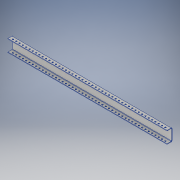
# Autodesk Inventor part: Intake front inner
Saved by Autodesk Inventor 2019 (Build 230136000, 136)
## iProperties
Created: 2018-11-07
Part Number: Intake front inner
Material: Aluminum 6061
Document SubType Name: Sheet Metal
Designer: woodk
Density: 2.7 g/cm^3
Sheet Metal Rule: Haakon
Appearance: Aluminum - Flat
Mass: 253.541 g
Surface Area: 982.103 cm^2
Volume: 93.904 cm^3
Author: woodk
Autodesk Inventor part; units mm, degrees
ref_plane "YZ Plane" through (0, 0, 0) normal (1, 0, 0) x (0, 1, 0)
ref_plane "XZ Plane" through (0, 0, 0) normal (0, 1, 0) x (-1, 0, 0)
ref_plane "XY Plane" through (0, 0, 0) normal (0, 0, 1) x (1, 0, 0)
sketch "Sketch1" plane through (0, 0, 0) normal (0, 0, 1) x (1, 0, 0)
  line L0 (0, 0) -> (609.6, 0)
  line L1 (609.6, 0) -> (609.6, 46.736)
  line L2 (609.6, 46.736) -> (0, 46.736)
  line L3 (0, 46.736) -> (0, 0)
  dimension "d0" = 46.736
  dimension "d1" = 609.6
  measures "d0" distance of L2.end L0.start
  measures "d1" distance of L0.start L0.end
extrude "Plate1" add sketch "Sketch1" along normal blind 2.032
sketch "Sketch2" plane through (0, 44.704, 0) normal (0, 1, 0) x (-1, 0, 0)
  line L0 (-609.6, 0) -> (0, 0)
  line L1 (0, 0) -> (0, 19.05)
  line L2 (0, 19.05) -> (-609.6, 19.05)
  line L3 (-609.6, 19.05) -> (-609.6, 0)
  constraints: 6 end point, 1 horizontal, 1 perpendicular, 1 vertical
edge flange "Flange1" height 19.05 angle 90 thickness 2.032 bend radius 1.27 thickness toward (0, 1, 0) relief tear relief width 2.032 relief depth 1.016 edges at (304.8, 46.736, 2.032) wall of the first edge with corners at (609.6, 44.704, 0) (0, 44.704, 0) (0, 44.704, 19.05) (609.6, 44.704, 19.05)
bend "Bend1"
corner "Corner1"
sketch "Sketch3" plane through (609.6, 2.032, 0) normal (0, -1, 0) x (1, 0, 0)
  line L0 (-609.6, 0) -> (0, 0)
  line L1 (0, 0) -> (0, 19.05)
  line L2 (0, 19.05) -> (-609.6, 19.05)
  line L3 (-609.6, 19.05) -> (-609.6, 0)
  constraints: 6 end point, 1 horizontal, 1 perpendicular, 1 vertical
edge flange "Flange2" height 19.05 angle 90 thickness 2.032 bend radius 1.27 thickness toward (0, -1, 0) relief tear relief width 2.032 relief depth 1.016 edges at (304.8, 0, 2.032) wall of the first edge with corners at (0, 2.032, 0) (609.6, 2.032, 0) (609.6, 2.032, 19.05) (0, 2.032, 19.05)
bend "Bend2"
corner "Corner2"
sketch "Sketch4" plane through (0, 46.736, 19.05) normal (0, 1, 0) x (1, 0, 0)
  line L0 (0, 0) -> (0, 15.748) projected
  line L1 (0, 19.05) -> (609.6, 19.05) projected
  point P0 (12.7, 6.35)
  dimension "d23" = 12.7
  dimension "d24" = 12.7
  measures "d23" distance from line of L0 point (12.7, 6.35)
  measures "d24" distance from line of L1 point (12.7, 6.35)
hole "Hole1" at (12.7, 46.736, 12.7) direction (0, -1, 0) diameter 4.9784 end through all
pattern_linear "Rectangular Pattern1" count 47 spacing 12.7 along (1, 0, 0) of "Hole1"
equation "\"d30\" = Thickness"
equation "\"d2\" = Thickness"
equation "\"d3\" = BendReliefWidth"
equation "\"d4\" = BendReliefDepth"
equation "\"d5\" = MinimumRemnant"
equation "\"d6\" = TransitionRadius"
equation "\"d9\" = BendRadius"
equation "\"d10\" = CornerReliefSize"
equation "\"d11\" = GapSize"
equation "\"d12\" = JacobiRadiusSize"
equation "\"d13\" = BendReliefWidth"
equation "\"d14\" = BendReliefDepth"
equation "\"d15\" = MinimumRemnant"
equation "\"d16\" = TransitionRadius"
equation "\"d19\" = BendRadius"
equation "\"d20\" = CornerReliefSize"
equation "\"d21\" = GapSize"
equation "\"d22\" = JacobiRadiusSize"
equation "\"BendReliefWidth\" = Thickness"
equation "\"BendReliefDepth\" = 0.5 * Thickness"
equation "\"CornerReliefSize\" = 4 * Thickness"
equation "\"MinimumRemnant\" = 2 * Thickness"
equation "\"TransitionRadius\" = BendRadius"
equation "\"JacobiRadiusSize\" = BendRadius"
equation "\"GapSize\" = Thickness"
equation "\"Thickness\" = 2.032"
equation "\"BendRadius\" = 1.27"
body "Solid1"
